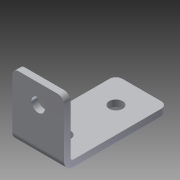
# Autodesk Inventor part: Chassis Bumper Mount - front and back
Saved by Autodesk Inventor 2013 (Build 170138000, 138)
## iProperties
Created: 2013-01-14
Part Number: Chassis Bumper Mount - front and back
Material: Aluminum 6061
Document SubType Name: Sheet Metal
Designer: Moses
Density: 2.71 g/cm^3
Mass: 16.1206 g
Surface Area: 45.8496 cm^2
Volume: 5.94855 cm^3
Sheet Metal Rule: Default
Author: Moses
Autodesk Inventor part; units mm, degrees
ref_plane "YZ Plane" through (0, 0, 0) normal (1, 0, 0) x (0, 1, 0)
ref_plane "XZ Plane" through (0, 0, 0) normal (0, 1, 0) x (-1, 0, 0)
ref_plane "XY Plane" through (0, 0, 0) normal (0, 0, 1) x (1, 0, 0)
sketch "Sketch1" plane through (0, 0, 0) normal (0, 1, 0) x (-1, 0, 0)
  line L0 (0, 0) -> (0, 50.8)
  line L1 (0, 50.8) -> (25.4, 50.8)
  line L2 (25.4, 50.8) -> (25.4, 0)
  line L3 (25.4, 0) -> (0, 0)
  circle A0 centre (12.7, 38.1) radius 3.302
  circle A1 centre (12.7, 12.7) radius 3.302
  line L4 (0, 25.4) -> (25.4, 25.4) construction
  line L5 (12.7, 38.1) -> (12.7, 12.7) construction
  point P0 (12.7, 25.4)
  dimension "d0" = 50.8
  dimension "d1" = 25.4
  dimension "d2" = 6.604
  dimension "d3" = 6.604
  dimension "d4" = 25.4
  measures "d0" distance of L0.start L0.end
  measures "d1" distance of L0.end L1.end
  measures "d2" diameter of A0
  measures "d3" diameter of A1
  measures "d4" distance of L5.start L5.end
extrude "Plate1" add sketch "Sketch1" along normal blind 3.175
sketch "Sketch2" plane through (0, 0, 47.625) normal (0, 0, 1) x (1, 0, 0)
  line L0 (-25.4, 0) -> (0, 0)
  line L1 (0, 0) -> (0, 31.75)
  line L2 (0, 31.75) -> (-25.4, 31.75)
  line L3 (-25.4, 31.75) -> (-25.4, 0)
  constraints: 6 end point, 1 horizontal, 1 perpendicular, 1 vertical
edge flange "Flange1" height 31.75 angle 90 thickness 3.175 bend radius 1.27 thickness toward (0, 0, 1) relief tear relief width 3.175 relief depth 1.5875 edges at (-12.7, 3.175, 50.8) wall of the first edge with corners at (-25.4, 0, 47.625) (0, 0, 47.625) (0, 31.75, 47.625) (-25.4, 31.75, 47.625)
bend "Bend1"
corner "Corner1"
sketch "Sketch3" plane through (-25.4, 31.75, 50.8) normal (0, 0, 1) x (1, 0, 0)
  line L0 (0, 0) -> (25.4, 0) projected
  circle A0 centre (12.7, -9.525) radius 3.302
  line L1 (25.4, -31.75) -> (0, -31.75) construction
  line L2 (12.7, 0) -> (12.7, -31.75) construction
  dimension "d19" = 6.604
  dimension "d21" = 22.225
  constraints: 2 end point, 2 midpoint, 1 centre point, 1 point on line
  measures "d19" diameter of A0
  measures "d21" distance from line of L1 A0.centre
extrude "Cut1" cut sketch "Sketch3" against normal blind 3.175
fillet "Corner Round1" radius 3.175 4 edges at (0, 31.75, 49.2125) (-25.4, 31.75, 49.2125) (0, 1.5875, 0) (-25.4, 1.5875, 0)
equation "\"d3\" = d2"
equation "\"d22\" = Thickness"
equation "\"d9\" = BendReliefWidth"
equation "\"d10\" = BendReliefDepth"
equation "\"d11\" = MinimumRemnant"
equation "\"d12\" = BendRadius"
equation "\"d16\" = CornerReliefSize"
equation "\"d17\" = GapSize"
equation "\"d18\" = JacobiRadiusSize"
equation "\"BendRadius\" = Thickness"
equation "\"BendReliefWidth\" = Thickness"
equation "\"BendReliefDepth\" = 0.5 * Thickness"
equation "\"CornerReliefSize\" = 4 * Thickness"
equation "\"MinimumRemnant\" = 2 * Thickness"
equation "\"TransitionRadius\" = BendRadius"
equation "\"JacobiRadiusSize\" = Thickness"
equation "\"GapSize\" = Thickness"
equation "\"d8\" = BendRadius"
equation "\"Thickness\" = 3.175"
body "Solid2"
